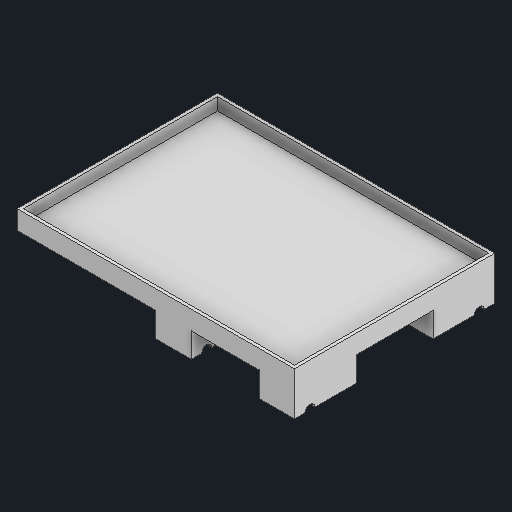
# Autodesk Inventor part: table_bed
Saved by Autodesk Inventor 2025 (Build 290162010, 162A)
## iProperties
Created: 2024-06-21
Part Number: table_bed
Material: Generic
Document SubType Name: Modeling
Designer: mihir
Density: 1 g/cm^3
Appearance: Default
Author: mihir
Autodesk Inventor part; units mm, degrees
ref_plane "YZ Plane" through (0, 0, 0) normal (1, 0, 0) x (0, 1, 0)
ref_plane "XZ Plane" through (0, 0, 0) normal (0, 1, 0) x (-1, 0, 0)
ref_plane "XY Plane" through (0, 0, 0) normal (0, 0, 1) x (1, 0, 0)
sketch "Sketch1" plane through (0, 0, 0) normal (0, 1, 0) x (-1, 0, 0)
  line L0 (0, 0) -> (180, 0)
  line L1 (180, 0) -> (180, -130)
  line L2 (180, -130) -> (0, -130)
  line L3 (0, -130) -> (0, 0)
  dimension "d0" = 130
  dimension "d1" = 180
  constraints: 8 end point, 2 parallel, 1 horizontal, 1 perpendicular
  measures "d0" distance of L2.end L0.start
  measures "d1" distance of L0.start L0.end
extrude "Extrusion1" add sketch "Sketch1" along normal blind 12.2
sketch "Sketch2" plane through (0, 12.2, 0) normal (0, 1, 0) x (1, 0, 0)
  line L0 (-178, 2) -> (-2, 2)
  line L1 (-2, 2) -> (-2, 128)
  line L2 (-2, 128) -> (-178, 128)
  line L3 (-178, 128) -> (-178, 2)
  line L4 (-180, 130) -> (-180, 0) projected
  line L5 (-180, 0) -> (0, 0) projected
  dimension "d4" = 2
  dimension "d5" = 2
  dimension "d6" = 176
  dimension "d7" = 126
  constraints: 8 end point, 2 parallel, 1 horizontal, 1 perpendicular
  measures "d4" distance between parallel lines of L4 L3
  measures "d5" distance between parallel lines of L5 L0
  measures "d6" distance of L0.start L0.end
  measures "d7" distance of L2.end L0.start
extrude "Extrusion2" cut sketch "Sketch2" against normal blind 8
sketch "Sketch3" plane through (0, 0, 0) normal (0, -1, 0) x (1, 0, 0)
  line L0 (0, 0) -> (-23, 0)
  line L1 (-23, 0) -> (-23, -40)
  line L2 (-23, -40) -> (0, -40)
  line L3 (0, -40) -> (0, 0)
  dimension "d10" = 23
  dimension "d11" = 40
  constraints: 8 end point, 2 parallel, 1 horizontal, 1 perpendicular
  measures "d10" distance of L1.end L2.end
  measures "d11" distance of L0.end L1.end
extrude "Extrusion3" add sketch "Sketch3" along normal blind 16
sketch "Sketch4" plane through (0, -16, 0) normal (0, -1, 0) x (1, 0, 0)
  line L0 (-1.5, -4) -> (-21.5, -4)
  line L1 (-21.5, -4) -> (-21.5, -10)
  line L2 (-21.5, -10) -> (-1.5, -10)
  line L3 (-1.5, -10) -> (-1.5, -4)
  line L4 (0, -40) -> (0, 0) projected
  line L5 (-1.5, -4) -> (0, -4) construction
  line L6 (0, 0) -> (-23, 0) construction
  dimension "d14" = 6
  dimension "d15" = 20
  dimension "d16" = 1.5
  dimension "d17" = 4
  constraints: 10 end point, 2 parallel, 2 perpendicular, 1 horizontal, 1 point on line
  measures "d14" distance of L2.end L0.start
  measures "d15" distance of L0.start L0.end
  measures "d16" distance between parallel lines of L4 L3
  measures "d17" distance between parallel lines of L6 L0
revolve "Revolution1" cut sketch "Sketch4" angle 360 about axis through (-21.5, -16, -10) along (1, 0, 0)
sketch "Sketch5" plane through (0, -16, 0) normal (0, -1, 0) x (1, 0, 0)
  line L0 (-23, -40) -> (0, -40) projected
  line L1 (-4.5, -22.5) -> (-18.5, -22.5) construction
  line L2 (-11.5, -22.5) -> (-11.5, -40) construction
  line L3 (0, 0) -> (-23, 0) projected
  dimension "d19" = 14
  dimension "d31" = 22.5
  constraints: 4 end point, 2 midpoint, 1 horizontal, 1 vertical
  measures "d19" distance of L1.end L1.start
  measures "d31" distance from line of L3 L1.start
hole "Hole1" at (-4.5, -16, -22.5) at (-18.5, -16, -22.5) direction (0, 1, 0) diameter 3 depth 16 tip angle 118
ref_plane "Work Plane1" through (-180, 12.2, -65) normal (0, 0, 1) x (1, 0, 0)
ref_plane "Work Plane2" through (-90, 0, -130) normal (1, 0, 0) x (0, 0, -1)
mirror "Mirror1" about plane through (-180, 12.2, -65) normal (0, 0, 1) of "Extrusion3", "Revolution1", "Hole1"
ref_plane "Work Plane3" through (-45, 0, -130) normal (1, 0, 0) x (0, 0, -1)
mirror "Mirror2" about plane through (-45, 0, -130) normal (1, 0, 0) of "Extrusion3", "Revolution1", "Hole1", "Mirror1"
sketch "Sketch6" plane through (0, 12.2, 0) normal (1, 0, 0) x (0, 0, -1)
  arc A0 (16, -28.2) -> (4, -28.2) centre (10, -28.2) ccw projected
  line L0 (4, -28.2) -> (16, -28.2) projected
  arc A1 (13.25, -28.2) -> (6.75, -28.2) centre (10, -28.2) ccw
  line L1 (6.75, -28.2) -> (13.25, -28.2)
  point P0 (0, -12.2)
  point P1 (6.75, -28.2)
  dimension "d28" = 3.25
  constraints: 2 end point, 2 point on circle, 1 centre point, 1 coincident, 1 collinear, 1 point on line
  measures "d28" radius of A1
extrude "Extrusion4" cut sketch "Sketch6" against normal up to surface (90 mm away) contours L0 A1
mirror "Mirror3" about plane through (-180, 12.2, -65) normal (0, 0, 1) of "Extrusion4"
equation "\"d0\" = table_bed_width"
equation "\"d1\" = table_bed_length"
equation "\"d2\" = table_bed_thickness"
equation "\"d4\" = table_bed_wall_thickness"
equation "\"d5\" = table_bed_wall_thickness"
equation "\"d6\" = table_bed_length - 2 * table_bed_wall_thickness"
equation "\"d7\" = table_bed_width - 2 * table_bed_wall_thickness"
equation "\"d8\" = table_bed_indent_depth"
equation "\"d10\" = table_bed_peg_width"
equation "\"d11\" = table_bed_peg_length"
equation "\"d12\" = table_bed_peg_height"
equation "\"d14\" = 0.5 * bearing_diameter"
equation "\"d15\" = bearing_length"
equation "\"d16\" = 0.5 * table_bed_peg_width - 0.5 * bearing_length"
equation "\"d19\" = screw_x"
equation "\"d31\" = screw_y"
equation "\"d21\" = screw_diameter"
equation "\"d28\" = 0.5 * rod_free_tolerance + 0.5 * rod_diameter"
equation "\"table_bed_width\" = 130"
equation "\"table_bed_length\" = 180"
equation "\"table_bed_thickness\" = 12.2"
equation "\"table_bed_indent_depth\" = 8"
equation "\"table_bed_wall_thickness\" = 2"
equation "\"screw_diameter\" = 3"
equation "\"table_bed_peg_length\" = 40"
equation "\"table_bed_peg_width\" = 23"
equation "\"table_bed_peg_height\" = 16"
equation "\"bearing_length\" = 20"
equation "\"bearing_diameter\" = 12"
equation "\"screw_x\" = 14"
equation "\"screw_y\" = 22.5"
equation "\"rod_diameter\" = 6"
equation "\"rod_free_tolerance\" = 0.5"
body "Solid1"
